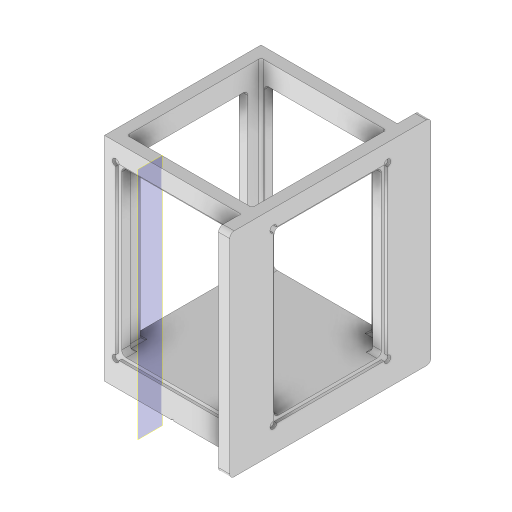
# Autodesk Inventor part: cuvette-w70mm-slide50x75mm-v1
Saved by Autodesk Inventor 2023 (Build 270158000, 158)
## iProperties
Created: 2025-09-30
Part Number: cuvette-w70mm-slide50x75mm-v1
Material: Generic
Document SubType Name: Modeling
Designer: N.Vladimirov
Density: 1 g/cm^3
Appearance: Default
Author: N.Vladimirov
Autodesk Inventor part; units mm, degrees
ref_plane "YZ Plane" through (0, 0, 0) normal (1, 0, 0) x (0, 1, 0)
ref_plane "XZ Plane" through (0, 0, 0) normal (0, 1, 0) x (-1, 0, 0)
ref_plane "XY Plane" through (0, 0, 0) normal (0, 0, 1) x (1, 0, 0)
sketch "Sketch1" plane through (0, 0, 0) normal (0, 0, 1) x (1, 0, 0)
  line L0 (30.5, -35) -> (-30.5, -35)
  line L1 (-30.5, -35) -> (-30.5, 35)
  line L2 (-30.5, 35) -> (30.5, 35)
  line L3 (30.5, 35) -> (30.5, -35)
  line L4 (30.5, -35) -> (-30.5, 35) construction
  line L5 (-30.5, -35) -> (30.5, 35) construction
  point P0 (0, 0)
  dimension "d0" = 61
  dimension "d1" = 70
  constraints: 12 end point, 2 midpoint, 2 parallel, 1 horizontal, 1 perpendicular
  measures "d0" distance of L1.end L2.end
  measures "d1" distance of L0.end L1.end
extrude "Extrusion1" add sketch "Sketch1" along normal blind 95.25
sketch "Sketch2" plane through (30.5, -35, 0) normal (1, 0, 0) x (0, 0, -1)
  line L0 (0, 0) -> (0, 70) projected
  line L1 (0, 70) -> (-95.25, 70) projected
  line L2 (-95.25, 0) -> (-95.25, 70) projected
  line L3 (0, 0) -> (-95.25, 0) projected
  line L4 (0, 70) -> (-95.25, 70) projected
  line L5 (-95.25, 70) -> (0, 70)
  line L6 (0, 70) -> (0, 80)
  line L7 (0, 80) -> (-95.25, 80)
  line L8 (-95.25, 80) -> (-95.25, 70)
  line L9 (-95.25, 70) -> (-95.25, 0) projected
  line L10 (-95.25, 0) -> (0, 0)
  line L11 (0, 0) -> (0, -10)
  line L12 (0, -10) -> (-95.25, -10)
  line L13 (-95.25, -10) -> (-95.25, 0)
  point P0 (0, 35)
  dimension "d4" = 10
  dimension "d5" = 10
  constraints: 16 end point, 4 parallel, 2 horizontal, 2 perpendicular, 1 point on line
  measures "d4" distance of L6.end L5.end
  measures "d5" distance of L10.end L11.end
extrude "Extrusion2" add sketch "Sketch2" along normal blind 5
sketch "Sketch12" plane through (35.5, -35, 0) normal (1, 0, 0) x (0, 0, -1)
  line L0 (-82.5, 9.5) -> (-9.5, 9.5)
  line L1 (-8, 11) -> (-8, 59)
  line L2 (-9.5, 60.5) -> (-82.5, 60.5)
  line L3 (-84, 59) -> (-84, 11)
  line L4 (-84, 9.5) -> (-8, 60.5) construction
  line L5 (-8, 9.5) -> (-84, 60.5) construction
  line L6 (-9.5, 57) -> (-9.5, 13)
  line L7 (-11.5, 11) -> (-80.5, 11)
  line L8 (-82.5, 13) -> (-82.5, 57)
  line L9 (-80.5, 59) -> (-11.5, 59)
  line L10 (0, -10) -> (0, 80) projected
  arc A0 (-9.5, 57) -> (-11.5, 59) centre (-11.5, 57) ccw
  arc A1 (-11.5, 11) -> (-9.5, 13) centre (-11.5, 13) ccw
  arc A2 (-82.5, 13) -> (-80.5, 11) centre (-80.5, 13) ccw
  arc A3 (-80.5, 59) -> (-82.5, 57) centre (-80.5, 57) ccw
  arc A4 (-8, 59) -> (-9.5, 60.5) centre (-8, 60.5) ccw
  arc A5 (-9.5, 9.5) -> (-8, 11) centre (-8, 9.5) ccw
  arc A6 (-82.5, 60.5) -> (-84, 59) centre (-84, 60.5) ccw
  arc A7 (-84, 11) -> (-82.5, 9.5) centre (-84, 9.5) ccw
  point P0 (0, 35)
  point P1 (-46, 35)
  point P2 (0, -8)
  point P3 (0, 78)
  dimension "d55" = 76
  dimension "d56" = 51
  dimension "d57" = 1.5
  dimension "d58" = 8
  dimension "d59" = 2
  dimension "d60" = 3
  dimension "d61" = 3
  dimension "d62" = 3
  dimension "d63" = 3
  constraints: 20 end point, 16 point on circle, 8 centre point, 8 tangent, 4 coincident, 4 parallel, 3 equal radius, 2 midpoint, 2 perpendicular, 1 horizontal
  measures "d55" distance of L5.end L4.end
  measures "d56" distance of L4.end L5.start
  measures "d57" distance between parallel lines of L1 L6
  measures "d58" distance between parallel lines of L1 L10
  measures "d59" radius of A0
  measures "d60" diameter of A4
  measures "d61" diameter of A5
  measures "d62" diameter of A6
  measures "d63" diameter of A7
sketch "Sketch13" plane through (-30.5, -35, 0) normal (-1, 0, 0) x (0, 0, 1)
  line L0 (8, 11) -> (8, 59) projected
  line L1 (9.5, 57) -> (9.5, 13) projected
  line L2 (82.5, 9.5) -> (9.5, 9.5) projected
  arc A0 (8, 11) -> (9.5, 9.5) centre (8, 9.5) ccw projected
  line L3 (11.5, 11) -> (80.5, 11) projected
  arc A1 (9.5, 13) -> (11.5, 11) centre (11.5, 13) ccw projected
  arc A2 (9.5, 60.5) -> (8, 59) centre (8, 60.5) ccw projected
  line L4 (9.5, 60.5) -> (82.5, 60.5) projected
  line L5 (80.5, 59) -> (11.5, 59) projected
  line L6 (84, 59) -> (84, 11) projected
  line L7 (82.5, 13) -> (82.5, 57) projected
  arc A3 (84, 59) -> (82.5, 60.5) centre (84, 60.5) ccw projected
  arc A4 (82.5, 9.5) -> (84, 11) centre (84, 9.5) ccw projected
  arc A5 (80.5, 11) -> (82.5, 13) centre (80.5, 13) ccw projected
  arc A6 (82.5, 57) -> (80.5, 59) centre (80.5, 57) ccw projected
  arc A7 (11.5, 59) -> (9.5, 57) centre (11.5, 57) ccw projected
  point P0 (0, 35)
extrude "Extrusion12" cut sketch "Sketch12" against normal through all contours L6 A1 L7 A2 L8 A3 L9 A0
ref_plane "LightSheet Plane1" through (-5.1, -35, 0) normal (-1, 0, 0) x (0, 0, 1)
sketch "Sketch15" plane through (-30.5, 35, 95.25) normal (0, 1, 0) x (1, 0, 0)
  line L0 (54.5, 11.25) -> (6.5, 11.25)
  line L1 (5, 12.75) -> (5, 85.75)
  line L2 (6.5, 87.25) -> (54.5, 87.25)
  line L3 (56, 85.75) -> (56, 12.75)
  line L4 (56, 11.25) -> (5, 87.25) construction
  line L5 (5, 11.25) -> (56, 87.25) construction
  line L6 (61, 95.25) -> (0, 95.25) projected
  line L7 (52.5, 85.75) -> (8.5, 85.75)
  line L8 (6.5, 83.75) -> (6.5, 14.75)
  line L9 (8.5, 12.75) -> (52.5, 12.75)
  line L10 (54.5, 14.75) -> (54.5, 83.75)
  arc A0 (8.5, 85.75) -> (6.5, 83.75) centre (8.5, 83.75) ccw
  arc A1 (54.5, 83.75) -> (52.5, 85.75) centre (52.5, 83.75) ccw
  arc A2 (52.5, 12.75) -> (54.5, 14.75) centre (52.5, 14.75) ccw
  arc A3 (6.5, 14.75) -> (8.5, 12.75) centre (8.5, 14.75) ccw
  arc A4 (6.5, 87.25) -> (5, 85.75) centre (5, 87.25) ccw
  arc A5 (56, 85.75) -> (54.5, 87.25) centre (56, 87.25) ccw
  arc A6 (54.5, 11.25) -> (56, 12.75) centre (56, 11.25) ccw
  arc A7 (5, 12.75) -> (6.5, 11.25) centre (5, 11.25) ccw
  point P0 (30.5, 95.25)
  point P1 (30.5, 49.25)
  dimension "d82" = 51
  dimension "d83" = 76
  dimension "d84" = 8
  dimension "d85" = 1.5
  dimension "d86" = 2
  dimension "d87" = 3
  dimension "d88" = 3
  dimension "d89" = 3
  dimension "d90" = 3
  constraints: 20 end point, 16 point on circle, 8 centre point, 8 tangent, 4 coincident, 4 parallel, 3 equal radius, 2 midpoint, 2 perpendicular, 1 horizontal
  measures "d82" distance of L4.end L5.end
  measures "d83" distance of L5.start L4.end
  measures "d84" distance between parallel lines of L2 L6
  measures "d85" distance between parallel lines of L2 L7
  measures "d86" radius of A0
  measures "d87" diameter of A4
  measures "d88" diameter of A5
  measures "d89" diameter of A6
  measures "d90" diameter of A7
extrude "Extrusion16" cut sketch "Sketch15" against normal through all contours A1 L10 A2 L9 A3 L8 A0 L7
sketch "Sketch16" plane through (-30.5, -35, 0) normal (0, -1, 0) x (1, 0, 0)
  line L0 (6.5, 8) -> (54.5, 8) projected
  arc A0 (5, 9.5) -> (6.5, 8) centre (5, 8) ccw projected
  line L1 (5, 82.5) -> (5, 9.5) projected
  arc A1 (54.5, 8) -> (56, 9.5) centre (56, 8) ccw projected
  line L2 (56, 9.5) -> (56, 82.5) projected
  arc A2 (56, 82.5) -> (54.5, 84) centre (56, 84) ccw projected
  line L3 (54.5, 84) -> (6.5, 84) projected
  arc A3 (6.5, 84) -> (5, 82.5) centre (5, 84) ccw projected
  point P0 (30.5, 0)
extrude "Extrusion17" cut sketch "Sketch16" against normal blind 1.2
sketch "Sketch17" plane through (0, 0, 0) normal (0, 0, -1) x (-1, 0, 0)
  line L0 (25.5, 30) -> (-30.5, 30)
  line L1 (-30.5, 30) -> (-30.5, -30)
  line L2 (-30.5, -30) -> (25.5, -30)
  line L3 (25.5, -30) -> (25.5, 30)
  line L4 (-30.5, 35) -> (30.5, 35) projected
  line L5 (30.5, 35) -> (30.5, -35) projected
  line L6 (30.5, -35) -> (-30.5, -35) projected
  line L7 (-30.5, 35) -> (-30.5, 45) projected
  point P0 (0, 0)
  dimension "d95" = 5
  dimension "d96" = 5
  dimension "d97" = 5
  dimension "d98" = 0
  constraints: 8 end point, 2 parallel, 1 horizontal, 1 perpendicular
  measures "d95" distance between parallel lines of L0 L4
  measures "d96" distance between parallel lines of L3 L5
  measures "d97" distance between parallel lines of L6 L2
  measures "d98" distance between parallel lines of L7 L1
extrude "Extrusion18" cut sketch "Sketch17" against normal up to surface (82.5 mm away)
fillet "Fillet2" radius 1 12 edges at (30.5, 26, 82.5) (26.25, 30, 82.5) (30.5, 30, 41.25) (30.5, -30, 41.25) (26.25, -30, 82.5) (30.5, -26, 82.5) (-25.5, -30, 41.25) (-25.5, 30, 41.25) (-25.5, -26, 82.5) (-25.5, 26, 82.5) (-23.75, 30, 82.5) (-23.75, -30, 82.5)
extrude "Extrusion19" cut sketch "Sketch15" against normal blind 1.2 contours L0 A7 L1 A4 L2 A5 L3 A6 | A1 L10 A2 L9 A3 L8 A0 L7
fillet "Fillet3" radius 2 4 edges at (33, 45, 0) (33, 45, 95.25) (33, -45, 0) (33, -45, 95.25)
extrude "Extrusion20" cut sketch "Sketch12" against normal blind 1.2 contours A7 L3 A6 L2 A4 L1 A5 L0 | L6 A1 L7 A2 L8 A3 L9 A0
extrude "Extrusion21" cut sketch "Sketch13" against normal blind 1.2 contours L0 A2 L4 A3 L6 A4 L2 A0 | A7 L5 A6 L7 A5 L3 A1 L1
sketch "Sketch18" plane through (0, 0, 95.25) normal (0, 0, 1) x (1, 0, 0)
  point P0 (0, 0)
  point P1 (0, 0)
  constraints: 1 coincident
hole "Hole2" at (0, 0, 95.25) direction (0, 0, -1) diameter 5.588 depth 10 tip angle 118 thread size "1/4-36 UNS" class "2B" standard "ANSI Unified Screw Threads"
sketch "Sketch19" plane through (-30.5, 35, 95.25) normal (0, 1, 0) x (1, 0, 0)
  circle A0 centre (30.5, 0) radius 0.5
  point P0 (30.5, 95.25)
  dimension "d116" = 1
  constraints: 1 centre point, 1 coincident
  measures "d116" diameter of A0
extrude "Extrusion22" cut sketch "Sketch19" against normal through all
body "Solid1"
